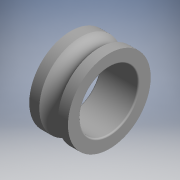
# Autodesk Inventor part: 6001JRX Inner Ring
Saved by Autodesk Inventor 2017.3 (Build 213256000, 256)
## iProperties
Part Number: 6001JRX Inner Ring
Material: Generic
Catalog Web Link: www.cadenas.de
Description: Open type ir-Deep Groove Ball Bearings
Vendor: NTN
Document SubType Name: Modeling
Designer: partserver
Manufacturer: NTN
Mass: 0.803082 g
Surface Area: 9.71663 cm^2
Volume: 0.803082 cm^3
Density: 1 g/cm^3
Appearance: PSOLRGB-192-192-192
Category: PARTsolutions
Company: NTN
Title: 6001JRX Inner Ring
Author: Cadenas PARTsolutions
Comments: Deep Groove Ball Bearings
PSOL_IDENT_0: {$CADENAS_DATA\23d-libs\ntn\ball_roller_bearings\deep_groove_bb\deep_groove_bb\6_types\dgbb_ir.prj},
PSOL_IDENT_1: 184 {VTYP=3D},{NB=6001JRX Inner Ring},{LINA=6001JRX Inner Ring},{NN=Open type ir},{DATE=12.08.2020 0
PSOL_IDENT_2: 2:23:39},{GEOMDATE=11.08.2020 08:58:19},{VERSION=},{LINEID=8990},{WBVAR=},{WBNUMERIC=}  {NB=6001JRX
PSOL_IDENT_3: Inner Ring},{LINA=6001JRX Inner Ring},{KT=DUMMY},{IDNR=},{SD=12},{D=28},{B=8},{R=0.3},{ORDER1=6001JR
PSOL_IDENT_4: X},{ORDER=6001JRX},{VERS=1},{CR=5.65},{COR=2.39},{CRF=MIN},{CORF=MIN},{LSG=26000},{LSO=30000},{MASS=
PSOL_IDENT_5: 0.021},{RNS=MIN},{LLH=MIN},{LLU=MIN},{ST=},{NCST=},{LTST=},{CST=},{SRG=},{SR=},{D1=26.44},{A=2.20},{
PSOL_IDENT_6: BA=0.90},{R0=0.30},{D2=32.7},{F=MIN},{DA1=},{DA2=},{DA=},{DX=MIN},{CY=},{CZ=},{RAS=},{RNAS=0.182},{X=
PSOL_IDENT_7: 8},{XVE=2}
NB: 6001JRX Inner Ring
NN: Open type ir
NT: Deep Groove Ball Bearings
NBSYN: $ORDER. Inner Ring
LINA: 6001JRX Inner Ring
CATALOG: NTN Corporation
SD: 12
D: 28
B: 8
R: 0.3
ORDER1: 6001JRX
ORDER: 6001JRX
VERS: 1
CR: 5.65
COR: 2.39
CRF: 0
CORF: 0
LSG: 26000
LSO: 30000
MASS: 0.021
RNS: 0
LLH: 0
LLU: 0
D1: 26.44
A: 2.2
BA: 0.9
R0: 0.3
D2: 32.7
F: 0
DX: 0
RNAS: 0.182
XVE: 2
SUPPLIER: NTN
ARTICLENO: 6001JRX Inner Ring
BOMINFO: 6001JRX Inner Ring
CREATOR: CADENAS GmbH
Autodesk Inventor part; units mm, degrees
sketch "Sketch_1" plane through (0, 0, 0) normal (0, 0, 1) x (1, 0, 0)
  line L0 (8, 0) -> (0, 0)
  arc A0 (0, 6.3) -> (0.3, 6) centre (0.3, 6.3) ccw
  line L1 (0.3, 6) -> (7.7, 6)
  arc A1 (7.7, 6) -> (8, 6.3) centre (7.7, 6.3) ccw
  line L2 (8, 6.3) -> (8, 8.56)
  line L3 (8, 8.56) -> (5.92, 8.56)
  arc A2 (2.08, 8.56) -> (5.92, 8.56) centre (4, 10) ccw
  line L4 (2.08, 8.56) -> (0, 8.56)
  line L5 (0, 8.56) -> (0, 6.3)
  constraints: 12 end point, 6 point on circle, 3 centre point
revolve "Revolution1" add sketch "Sketch_1" angle 360 about axis through (8, 0, 0) along (1, 0, 0)
ref_plane "dgbb_ir_XY" through (0, 0, 0) normal (1, 0, 0) x (0, 0, -1)
ref_plane "dgbb_ir_YZ" through (0, 0, 0) normal (0, 0, -1) x (0, 1, 0)
ref_plane "dgbb_ir_ZX" through (0, 0, 0) normal (0, 1, 0) x (1, 0, 0)
body "Solid1"
